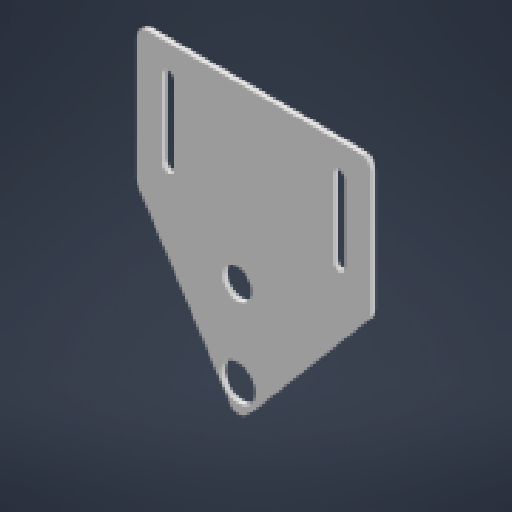
# Autodesk Inventor part: Part21
Saved by Autodesk Inventor 2023.2 (Build 272271000, 271)
## iProperties
Created: 2023-03-19
Part Number: Part21
Material: Generic
Document SubType Name: Modeling
Designer: Liam
Density: 1 g/cm^3
Appearance: Default
Author: Liam
Autodesk Inventor part; units mm, degrees
ref_plane "YZ Plane" through (0, 0, 0) normal (1, 0, 0) x (0, 1, 0)
ref_plane "XZ Plane" through (0, 0, 0) normal (0, 1, 0) x (-1, 0, 0)
ref_plane "XY Plane" through (0, 0, 0) normal (0, 0, 1) x (1, 0, 0)
sketch "Sketch1" plane through (0, 0, 0) normal (0, 0, 1) x (1, 0, 0)
  circle A0 centre (-0.2682, 25.3986) radius 2.0955
  circle A1 centre (0, 0) radius 5.2 projected
  line L0 (-19.0905, 68.1502) -> (-19.0905, 45.2902)
  line L1 (-22.4814, 68.1502) -> (-22.4814, 45.2902)
  line L2 (28.3186, 68.1502) -> (28.3186, 45.2902)
  line L3 (31.7095, 68.1502) -> (31.7095, 45.2902)
  arc A2 (-19.0905, 68.1502) -> (-22.4814, 68.1502) centre (-20.7859, 68.1502) ccw
  arc A3 (-22.4814, 45.2902) -> (-19.0905, 45.2902) centre (-20.7859, 45.2902) ccw
  arc A4 (31.7095, 68.1502) -> (28.3186, 68.1502) centre (30.0141, 68.1502) ccw
  arc A5 (28.3186, 45.2902) -> (31.7095, 45.2902) centre (30.0141, 45.2902) ccw
  line L4 (-22.4814, 56.7202) -> (-30.1014, 56.7202)
  line L5 (-30.1014, 56.7202) -> (-30.1014, 73.8652)
  line L6 (31.7095, 56.7202) -> (39.3295, 56.7202)
  line L7 (39.3295, 56.7202) -> (39.3295, 73.8652)
  line L8 (36.1545, 77.0402) -> (-26.9264, 77.0402)
  line L9 (-30.1014, 56.7202) -> (-30.1014, 37.3371)
  line L10 (39.3295, 56.7202) -> (39.3295, 37.5617)
  line L11 (0, 0) -> (0, -10.16)
  line L12 (-2.3266, -6.5613) -> (-29.5927, 35.6134)
  line L13 (2.7652, -6.8864) -> (38.58, 35.5129)
  arc A6 (-30.1014, 37.3371) -> (-29.5927, 35.6134) centre (-26.9264, 37.3371) ccw
  arc A7 (-26.9264, 77.0402) -> (-30.1014, 73.8652) centre (-26.9264, 73.8652) ccw
  arc A8 (39.3295, 73.8652) -> (36.1545, 77.0402) centre (36.1545, 73.8652) ccw
  arc A9 (38.58, 35.5129) -> (39.3295, 37.5617) centre (36.1545, 37.5617) ccw
  arc A10 (-2.3266, -6.5613) -> (2.7652, -6.8864) centre (0.3398, -4.8376) ccw
  circle A11 centre (-8.0859, 47.3249) radius 2.1844 projected
  circle A12 centre (17.3141, 47.3249) radius 2.1844 projected
  point P0 (0, 0)
  point P1 (-30.1014, 77.0402)
  point P2 (-30.1014, 36.4002)
  point P3 (39.3295, 36.4002)
  dimension "d5" = 7.62
  dimension "d6" = 20.32
  dimension "d7" = 7.62
  dimension "d8" = 20.32
  dimension "d9" = 20.32
  dimension "d10" = 10.16
  dimension "d11" = 3.175
  dimension "d12" = 4.191
  constraints: 28 end point, 18 point on circle, 18 tangent, 10 centre point, 9 vertical, 8 point on line, 4 equal radius, 2 horizontal, 2 midpoint, 1 perpendicular
  measures "d5" distance of L4.start L4.end
  measures "d6" distance of L4.end point (-30.101, 77.04)
  measures "d7" distance of L6.start L6.end
  measures "d8" distance of L4.end point (-30.101, 36.4)
  measures "d9" distance of L6.end point (39.33, 36.4)
  measures "d10" distance of L11.start L11.end
  measures "d11" radius of A6
  measures "d12" diameter of A0
extrude "Extrusion1" add sketch "Sketch1" along normal blind 1.524
body "Solid1"
